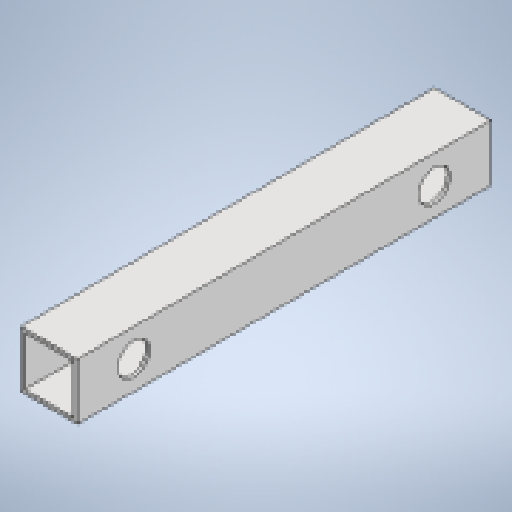
# Autodesk Inventor part: TZS 1663 FDS 940 way tube 3
Saved by Autodesk Inventor 2025.1 (Build 291241020, 241B)
## iProperties
Created: 2025-06-24
Part Number: TZS 1663 FDS 940 way tube 3
Material: Stainless Steel
Document SubType Name: Modeling
Designer: admin
Mass: 1762.25 g
Surface Area: 2283.33 cm^2
Volume: 220.281 cm^3
Density: 8 g/cm^3
Sheet Metal Rule: AISI304 2mm Die16
Sheet Metal Width: 0.000 mm
Sheet Metal Length: 0.000 mm
Sheet Metal Area: 0.000 mm^2
Appearance: Default
Author: user
Autodesk Inventor part; units mm, degrees
ref_plane "YZ Plane" through (0, 0, 0) normal (1, 0, 0) x (0, 1, 0)
ref_plane "XZ Plane" through (0, 0, 0) normal (0, 1, 0) x (-1, 0, 0)
ref_plane "XY Plane" through (0, 0, 0) normal (0, 0, 1) x (1, 0, 0)
sketch "Sketch9" plane through (0, 0, 0) normal (0, 1, 0) x (-1, 0, 0)
  line L0 (15, 15) -> (-15, 15)
  line L1 (-15, 15) -> (-15, -15)
  line L2 (-15, -15) -> (15, -15)
  line L3 (15, -15) -> (15, 15)
  line L4 (15, 15) -> (-15, -15) construction
  line L5 (-15, 15) -> (15, -15) construction
  line L6 (-13, 13) -> (13, 13)
  line L7 (13, 13) -> (13, -13)
  line L8 (13, -13) -> (-13, -13)
  line L9 (-13, -13) -> (-13, 13)
  point P0 (0, 0)
  dimension "d172" = 30
  dimension "d173" = 30
  dimension "d174" = 2
  constraints: 20 end point, 4 parallel, 2 midpoint, 2 perpendicular, 1 horizontal, 3 other
  measures "d172" distance of L2.end L1.end
  measures "d173" distance of L0.end L1.end
  measures "d174" distance between parallel lines of L0 L6
extrude "Extrusion3" add sketch "Sketch9" against normal blind 220
sketch "Sketch10" plane through (0, 0, 0) normal (1, 0, 0) x (0, 1, 0)
  line L0 (0, 15) -> (0, -15) construction
  line L1 (0, 15) -> (-220, 15) construction
  line L2 (-220, -15) -> (-220, 15) construction
  line L3 (0, -15) -> (-220, -15) construction
  line L4 (-68.5, 8.5) -> (-51.5, 8.5)
  line L5 (-51.5, 8.5) -> (-51.5, -8.5)
  line L6 (-51.5, -8.5) -> (-68.5, -8.5)
  line L7 (-68.5, -8.5) -> (-68.5, 8.5)
  line L8 (-68.5, 8.5) -> (-51.5, -8.5) construction
  line L9 (-51.5, 8.5) -> (-68.5, -8.5) construction
  line L10 (-198.5, 8.5) -> (-181.5, 8.5)
  line L11 (-181.5, 8.5) -> (-181.5, -8.5)
  line L12 (-181.5, -8.5) -> (-198.5, -8.5)
  line L13 (-198.5, -8.5) -> (-198.5, 8.5)
  line L14 (-198.5, 8.5) -> (-181.5, -8.5) construction
  line L15 (-181.5, 8.5) -> (-198.5, -8.5) construction
  line L16 (-428.5, 8.5) -> (-411.5, 8.5)
  line L17 (-411.5, 8.5) -> (-411.5, -8.5)
  line L18 (-411.5, -8.5) -> (-428.5, -8.5)
  line L19 (-428.5, -8.5) -> (-428.5, 8.5)
  line L20 (-428.5, 8.5) -> (-411.5, -8.5) construction
  line L21 (-411.5, 8.5) -> (-428.5, -8.5) construction
  circle A0 centre (-470, 0) radius 8.5
  line L22 (0, 0) -> (30, 0)
  circle A1 centre (-60, 0) radius 8.5
  circle A2 centre (-190, 0) radius 8.5
  circle A3 centre (-420, 0) radius 8.5
  dimension "d177" = 17
  dimension "d178" = 17
  dimension "d181" = 30
  dimension "d182" = 90
  dimension "d183" = 220
  dimension "d184" = 450
  dimension "d185" = 500
  dimension "d186" = 17
  constraints: 38 end point, 7 midpoint, 6 parallel, 4 centre point, 4 horizontal, 4 horizontal alignment, 3 coincident, 3 equal length, 3 perpendicular, 3 tangent, 1 point on line
  measures "d177" distance of L4.start L4.end
  measures "d178" distance of L4.end L5.end
  measures "d181" distance of L22.start L22.end
  measures "d182" distance of point (-60, 0) L22.end
  measures "d183" distance of point (-190, 0) L22.end
  measures "d184" distance of L22.end point (-420, 0)
  measures "d185" distance of L22.end A0.centre
  measures "d186" diameter of A0
extrude "Extrusion4" cut sketch "Sketch10" along normal through all contours A1 | A2
body "Solid4"
